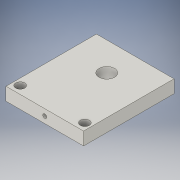
# Autodesk Inventor part: Grundplatte.0006
Saved by Autodesk Inventor 2018.3 (Build 223284000, 284)
## iProperties
Created: 2019-11-28
Material: Stahl, unlegiert
Document SubType Name: Modeling
Designer: bauermeisterdi
Density: 7.85 g/cm^3
Appearance: Stahl
Description: Grundplatte
Werkstoff: S235JRC+C
Author: bauermeisterdi
Autodesk Inventor part; units mm, degrees
ref_plane "YZ Plane" through (0, 0, 0) normal (1, 0, 0) x (0, 1, 0)
ref_plane "XZ Plane" through (0, 0, 0) normal (0, 1, 0) x (-1, 0, 0)
ref_plane "XY Plane" through (0, 0, 0) normal (0, 0, 1) x (1, 0, 0)
sketch "Skizze_Grundkörper" plane through (0, 0, 0) normal (0, 0, 1) x (1, 0, 0)
  line L0 (-42, 0) -> (42, 0) projected
  line L1 (0, -280) -> (0, 280) projected
  line L2 (30, -35) -> (-30, -35)
  line L3 (-30, -35) -> (-30, 35)
  line L4 (-30, 35) -> (30, 35)
  line L5 (30, 35) -> (30, -35)
  line L6 (30, -35) -> (-30, 35) construction
  line L7 (-30, -35) -> (30, 35) construction
  point P0 (0, 0)
  dimension "Breite" = 60
  dimension "Länge" = 70
  constraints: 12 end point, 2 midpoint, 2 parallel, 1 horizontal, 1 perpendicular
  measures "Breite" distance of L3.end L4.end
  measures "Länge" distance of L4.end L2.start
extrude "Grundkörper" add sketch "Skizze_Grundkörper" along normal mid plane 10
sketch "Skizze_Bohrung_12_mm" plane through (0, 0, 5) normal (0, 0, 1) x (1, 0, 0)
  line L0 (-42, 0) -> (42, 0) projected
  line L1 (0, -280) -> (0, 280) projected
  line L2 (-30, -35) -> (30, -35) projected
  line L3 (30, -35) -> (30, 35) projected
  line L4 (30, 35) -> (-30, 35) projected
  line L5 (-30, 35) -> (-30, -35) projected
  point P0 (0, 0)
  point P1 (0, 13)
  dimension "Bo_12_Abstand" = 48
  constraints: 1 point on line
  measures "Bo_12_Abstand" distance from line of point (0, 13) L2
hole "Bohrung_12_mm" at (0, 13, 5) direction (0, 0, -1) diameter 12 end through all
sketch "Skizze_7_mm" plane through (0, 0, 5) normal (0, 0, 1) x (1, 0, 0)
  line L0 (-42, 0) -> (42, 0) projected
  line L1 (0, -280) -> (0, 280) projected
  circle A0 centre (0, 13) radius 6 projected
  line L2 (-30, -35) -> (30, -35) projected
  line L3 (30, -35) -> (30, 35) projected
  line L4 (30, 35) -> (-30, 35) projected
  line L5 (-30, 35) -> (-30, -35) projected
  point P0 (0, 0)
  point P1 (-25, -29)
  point P2 (25, -29)
  dimension "Bo_7_Abstand" = 50
  dimension "Bo_7_Randabstand" = 6
  constraints: 1 symmetric about line
  measures "Bo_7_Abstand" distance of point (25, -29) point (-25, -29)
  measures "Bo_7_Randabstand" distance from line of point (25, -29) L2
hole "Bohrung_7_mm" at (-25, -29, 5) at (25, -29, 5) direction (0, 0, -1) diameter 7 end through all
sketch "Skizze_Bohrung_3_mm_unten" plane through (-30, -35, 5) normal (0, -1, 0) x (1, 0, 0)
  point P0 (30, -5)
  point P1 (30, -5)
  constraints: 1 coincident
hole "Bohrung_3_mm_unten" at (0, -35, 0) direction (0, 1, 0) diameter 3 depth 15 tip angle 118
sketch "Skizze_Bohrung_3_mm_oben" plane through (-30, 35, 5) normal (0, 1, 0) x (1, 0, 0)
  line L0 (0, 0) -> (0, 10) projected
  line L1 (60, 0) -> (0, 0) projected
  line L2 (60, 0) -> (60, 10) projected
  line L3 (0, 10) -> (60, 10) projected
  line L4 (-12, 5) -> (72, 5) projected
  line L5 (30, 12) -> (30, -2) projected
  point P0 (30, 5)
  point P1 (5, 5)
  point P2 (55, 5)
  dimension "d28" = 50
  constraints: 2 point on line, 1 symmetric about line
  measures "d28" distance of point (55, 5) point (5, 5)
hole "Bohrung_3_mm_oben" at (-25, 35, 0) at (25, 35, 0) direction (0, -1, 0) diameter 3 depth 15 tip angle 118
